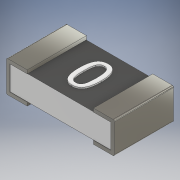
# Autodesk Inventor part: 21-1001
Saved by Autodesk Inventor 2018 (Build 220112000, 112)
## iProperties
Created: 2019-09-21
Part Number: 21-1001
Material: Copper
Document SubType Name: Modeling
Designer: Bradley
Density: 8.94 g/cm^3
Appearance: Smooth - White
Author: Bradley
Autodesk Inventor part; units mm, degrees
ref_plane "YZ Plane" through (0, 0, 0) normal (1, 0, 0) x (0, 1, 0)
ref_plane "XZ Plane" through (0, 0, 0) normal (0, 1, 0) x (-1, 0, 0)
ref_plane "XY Plane" through (0, 0, 0) normal (0, 0, 1) x (1, 0, 0)
sketch "Sketch1" plane through (0, 0, 0) normal (0, 1, 0) x (-1, 0, 0)
  line L0 (0.725, 0.175) -> (-0.725, 0.175)
  line L1 (-0.725, 0.175) -> (-0.725, -0.175)
  line L2 (-0.725, -0.175) -> (0.725, -0.175)
  line L3 (0.725, -0.175) -> (0.725, 0.175)
  line L4 (0.475, 0.175) -> (0.475, 0.225)
  line L5 (0.475, 0.225) -> (0.775, 0.225)
  line L6 (0.775, 0.225) -> (0.775, -0.225)
  line L7 (0.775, -0.225) -> (0.475, -0.225)
  line L8 (0.475, -0.225) -> (0.475, -0.175)
  line L9 (-0.475, 0.175) -> (-0.475, 0.225)
  line L10 (-0.475, 0.225) -> (-0.775, 0.225)
  line L11 (-0.775, 0.225) -> (-0.775, -0.225)
  line L12 (-0.775, -0.225) -> (-0.475, -0.225)
  line L13 (-0.475, -0.175) -> (-0.475, -0.225)
  line L14 (0.475, 0.175) -> (-0.475, 0.175)
  point P0 (0, 0)
  point P1 (0, 0.175)
  point P2 (0.725, 0)
  dimension "d0" = 1.55
  dimension "d1" = 0.05
  dimension "d2" = 0.05
  dimension "d3" = 0.45
  dimension "d4" = 0.3
  constraints: 30 end point, 12 point on line, 7 perpendicular, 3 collinear, 3 midpoint, 2 parallel, 1 horizontal, 1 horizontal alignment, 1 vertical, 1 vertical alignment
  measures "d0" distance between parallel lines of L11 L6
  measures "d1" distance of L7.end L8.end
  measures "d2" distance between parallel lines of L6 L3
  measures "d3" distance of L5.end L6.end
  measures "d4" distance of L6.end L7.end
extrude "Extrusion1" add sketch "Sketch1" along normal mid plane 0.85 contours L0 L4 L5 L6 L7 L8 L2 L3 | L0 L1 L2 L13 L12 L11 L10 L9
extrude "Extrusion2" add sketch "Sketch1" along normal mid plane 0.84 contours L3 L2 L1 L0
sketch "Sketch2" plane through (-0.475, -0.42, 0.175) normal (0, 0, 1) x (1, 0, 0)
  line L0 (0, 0) -> (0, 0.84) projected
  line L1 (0.95, 0) -> (0, 0) projected
  line L2 (0.95, 0) -> (0.95, 0.84) projected
  line L3 (0, 0.84) -> (0.95, 0.84) projected
  line L4 (0, 0.42) -> (0.95, 0.42) construction
  spline S0 degree 2 poles (0.635, 0.42) (0.635, 0.2855) (0.5568, 0.1595) (0.4754, 0.1595) knots 0 0 0 1 2 2 2
  spline S1 degree 2 poles (0.4754, 0.1595) (0.3927, 0.1595) (0.3154, 0.2879) (0.3154, 0.4196) knots 0 0 0 1 2 2 2
  spline S2 degree 2 poles (0.3154, 0.4196) (0.3154, 0.5549) (0.3936, 0.6801) (0.4754, 0.6801) knots 0 0 0 1 2 2 2
  spline S3 degree 2 poles (0.4754, 0.6801) (0.5577, 0.6801) (0.635, 0.5505) (0.635, 0.42) knots 0 0 0 1 2 2 2
  spline S4 degree 2 poles (0.5491, 0.2676) (0.5589, 0.2924) (0.567, 0.3685) (0.567, 0.42) knots 0 0 0 1 2 2 2
  spline S5 degree 2 poles (0.567, 0.42) (0.567, 0.4715) (0.5589, 0.5472) (0.5487, 0.5728) knots 0 0 0 1 2 2 2
  spline S6 degree 2 poles (0.5487, 0.5728) (0.5386, 0.5983) (0.5034, 0.6246) (0.4754, 0.6246) knots 0 0 0 1 2 2 2
  spline S7 degree 2 poles (0.4754, 0.6246) (0.4474, 0.6246) (0.4114, 0.5983) (0.4009, 0.5719) knots 0 0 0 1 2 2 2
  spline S8 degree 2 poles (0.4009, 0.5719) (0.3907, 0.5464) (0.3834, 0.4686) (0.3834, 0.4196) knots 0 0 0 1 2 2 2
  spline S9 degree 2 poles (0.3834, 0.4196) (0.3834, 0.3669) (0.3899, 0.2964) (0.4004, 0.2689) knots 0 0 0 1 2 2 2
  spline S10 degree 2 poles (0.4004, 0.2689) (0.4102, 0.2429) (0.4462, 0.215) (0.4754, 0.215) knots 0 0 0 1 2 2 2
  spline S11 degree 2 poles (0.4754, 0.215) (0.503, 0.215) (0.539, 0.2413) (0.5491, 0.2676) knots 0 0 0 1 2 2 2
  point P0 (0.475, 0.42)
  constraints: 2 end point, 2 midpoint, 1 horizontal
extrude "Extrusion3" add sketch "Sketch2" along normal blind 0.02 contours S0 S1 S2 S3
fillet "Fillet1" radius 0.02 4 edges at (-0.775, 0, 0.225) (-0.775, 0, -0.225) (0.775, 0, 0.225) (0.775, 0, -0.225)
equation "\"d2\" = d1"
body "Solid1"
